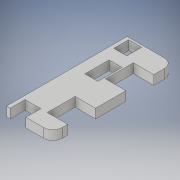
# Autodesk Inventor part: Charger_support
Saved by Autodesk Inventor 2017 (Build 210142000, 142)
## iProperties
Created: 2018-06-25
Part Number: Charger_support
Material: Generic
Document SubType Name: Modeling
Designer: Arthur
Density: 1 g/cm^3
Appearance: Default
Author: Arthur
Autodesk Inventor part; units mm, degrees
ref_plane "YZ Plane" through (0, 0, 0) normal (1, 0, 0) x (0, 1, 0)
ref_plane "XZ Plane" through (0, 0, 0) normal (0, 1, 0) x (-1, 0, 0)
ref_plane "XY Plane" through (0, 0, 0) normal (0, 0, 1) x (1, 0, 0)
sketch "Sketch1" plane through (0, 0, 0) normal (0, 1, 0) x (-1, 0, 0)
  line L0 (-14, 34.5) -> (11, 34.5)
  line L1 (11, 34.5) -> (11, -30.5)
  line L2 (11, -30.5) -> (-14, -30.5)
  line L3 (-14, -30.5) -> (-14, 34.5)
  dimension "d0" = 25
  dimension "d1" = 65
  constraints: 8 end point, 2 parallel, 1 horizontal, 1 perpendicular
  measures "d0" distance of L1.end L2.end
  measures "d1" distance of L0.end L1.end
extrude "Extrusion1" add sketch "Sketch1" along normal blind 5
fillet "Fillet1" radius 5 2 edges at (14, 2.5, 34.5) (14, 2.5, -30.5)
sketch "Sketch2" plane through (0, 5, 0) normal (0, 1, 0) x (1, 0, 0)
  line L0 (-9, -34.5716) -> (-9, -26.4716)
  line L1 (-9, -26.4716) -> (-0.5, -26.4716)
  line L2 (-0.5, -26.4716) -> (-0.5, -34.5716)
  line L3 (-0.5, -34.5716) -> (-9, -34.5716)
  point P0 (0, 0)
  point P1 (-11, -34.5)
  dimension "d6" = 8.1
  dimension "d7" = 8.5
  constraints: 8 end point, 2 perpendicular
  measures "d6" distance of L0.start L0.end
  measures "d7" distance of L0.end L1.end
extrude "Extrusion2" cut sketch "Sketch2" against normal through all
sketch "Sketch3" plane through (0, 5, 0) normal (0, 1, 0) x (1, 0, 0)
  line L0 (14, -26.5199) -> (3, -26.5199)
  line L1 (3, -26.5199) -> (3, -11.5199)
  line L2 (3, -11.5199) -> (14, -11.5199)
  line L3 (14, -11.5199) -> (14, -26.5199)
  line L4 (14, 4.8512) -> (3, 4.8512)
  line L5 (3, 4.8512) -> (3, 19.8512)
  line L6 (3, 19.8512) -> (14, 19.8512)
  line L7 (14, 19.8512) -> (14, 4.8512)
  point P0 (0, 0)
  dimension "d12" = 11
  dimension "d13" = 15
  dimension "d22" = 11
  dimension "d23" = 15
  constraints: 16 end point, 4 parallel, 2 horizontal, 2 perpendicular
  measures "d12" distance of L1.end L2.end
  measures "d13" distance of L0.end L1.end
  measures "d22" distance of L5.end L7.start
  measures "d23" distance of L4.end L5.end
extrude "Extrusion3" cut sketch "Sketch3" against normal through all
sketch "Sketch4" plane through (0, 5, 0) normal (0, 1, 0) x (1, 0, 0)
  line L0 (14, 4.8512) -> (3, 4.8512) projected
  line L1 (3, 19.8512) -> (3, 4.8512) projected
  line L2 (2.1235, 14.6407) -> (-4.8765, 14.6407)
  line L3 (-4.8765, 14.6407) -> (-4.8765, 1.6407)
  line L4 (-4.8765, 1.6407) -> (2.1235, 1.6407)
  line L5 (2.1235, 1.6407) -> (2.1235, 14.6407)
  line L6 (-11, 30.5) -> (-11, -34.5) projected
  line L7 (-9, 29.3191) -> (-2, 29.3191)
  line L8 (-2, 29.3191) -> (-2, 21.3191)
  line L9 (-2, 21.3191) -> (-9, 21.3191)
  line L10 (-9, 21.3191) -> (-9, 29.3191)
  point P0 (0, 0)
  dimension "d29" = 7
  dimension "d30" = 13
  dimension "d33" = 7
  dimension "d34" = 8
  constraints: 16 end point, 4 parallel, 2 horizontal, 2 perpendicular
  measures "d29" distance of L4.end L3.end
  measures "d30" distance of L3.end L2.end
  measures "d33" distance of L8.end L9.end
  measures "d34" distance of L7.end L8.end
extrude "Extrusion4" cut sketch "Sketch4" against normal through all
body "Solid1"
